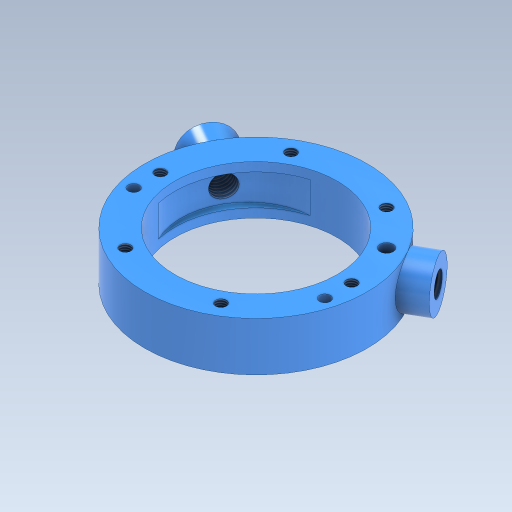
# Autodesk Inventor part: Pump-Motor-CW-Rotation:M Case
Saved by Autodesk Inventor 2024.2 (Build 282272000, 272)
## iProperties
Created: 2025-06-16
Material: Aluminum 6061-AHC
Document SubType Name: Modeling
Density: 2.7 g/cm^3
Appearance: Cyan
Designer: cw
Author: cw
Autodesk Inventor part; units mm, degrees
note: some values were not read from the file. Chosen so that the rebuilt part matches the saved one: direction of "Hole2".
ref_plane "YZ Plane" through (0, 0, 0) normal (1, 0, 0) x (0, 1, 0)
ref_plane "XZ Plane" through (0, 0, 0) normal (0, 1, 0) x (-1, 0, 0)
ref_plane "XY Plane" through (0, 0, 0) normal (0, 0, 1) x (1, 0, 0)
sketch "Sketch1" plane through (0, 0, 0) normal (0, 0, 1) x (1, 0, 0)
  circle A0 centre (0, 0) radius 50
  circle A1 centre (0, 0) radius 36.5
  dimension "d0" = 100
  dimension "d3" = 73
  constraints: 2 centre point, 2 coincident
  measures "d0" diameter of A0
  measures "d3" diameter of A1
extrude "Extrusion1" add sketch "Sketch1" along normal mid plane 22
sketch "Sketch2" plane through (0, 0, 0) normal (0, 0, 1) x (1, 0, 0)
  line L0 (0, 0) -> (51.961524, 30)
  line L1 (51.961524, 30) -> (57.461524, 20.473721)
  line L2 (57.461524, 20.473721) -> (47.740384, 14.861217)
  circle A0 centre (0, 0) radius 50 construction
  line L3 (47.740384, 14.861217) -> (42.240384, 24.387497)
  line L4 (-72.00542, 0) -> (82.032521, 0) construction
  dimension "d4" = 30
  dimension "d5" = 60
  dimension "d6" = 22
  constraints: 8 end point, 3 perpendicular, 1 point on line, 2 other
  measures "d4" angle of L4 L0
  measures "d5" distance from line of L1 L0.start
  measures "d6" diameter of L2 L0
revolve "Revolution1" add sketch "Sketch2" angle 360 about axis through (0, 0, 0) along (0.8660254, 0.5, 0)
mirror "Mirror1" about plane through (0, 0, 0) normal (1, 0, 0) of "Revolution1"
sketch "Sketch3" plane through (51.961524, 30, 0) normal (0.8660254, 0.5, 0) x (0, 0, -1)
  point P0 (0, 0)
hole "Hole1" at (51.961524, 30, 0) direction (-0.8660254, -0.5, 0) diameter 10.106 depth 32.3 tip angle 118 thread size "M12x1.75" class "6H" standard "ISO Metric profile"
sketch "Sketch4" plane through (0, 0, 0) normal (0, 0, 1) x (1, 0, 0)
  line L0 (0, 0) -> (-51.961524, 30) construction
  line L1 (-46.461524, 39.526279) -> (-57.461524, 20.473721) construction
  circle A0 centre (0, 0) radius 36.5
  arc A1 (-10.556856, 34.939988) -> (-35.537346, -8.327488) centre (-8.660254, 5) ccw
  dimension "d15" = 30
  dimension "d16" = 10
  constraints: 4 point on circle, 2 end point, 1 centre point, 1 midpoint, 1 point on line
  measures "d15" radius of A1
  measures "d16" distance of L0.start A1.centre
extrude "Extrusion2" cut sketch "Sketch4" along normal mid plane 14 contours A0 A1
sketch "Sketch5" plane through (-51.961524, 30, 0) normal (-0.8660254, 0.5, 0) x (0, 0, 1)
  point P0 (0, 0)
hole "Hole2" at (-51.961524, 30, 0) direction (0.8660254, -0.5, 0) diameter 10.106 end up to surface thread size "M12x1.75" class "6H" standard "ISO Metric profile"
sketch "Sketch6" plane through (0, 0, -11) normal (0, 0, -1) x (-1, 0, 0)
  circle A0 centre (0, 0) radius 43 construction
  point P0 (-43, 0)
  dimension "d26" = 86
  constraints: 2 horizontal alignment, 1 coincident, 2 other
hole "Hole3" at (43, 0, -11) direction (0, 0, 1) diameter 4.917 end through all thread size "M6x1" class "6H" standard "ISO Metric profile"
pattern_circular "Circular Pattern1" count 6 over 360 about axis through (0, 0, 0) along (0, 0, 1) of "Hole3"
sketch "Sketch7" plane through (0, 0, -11) normal (0, 0, -1) x (-1, 0, 0)
  circle A0 centre (43, 0) radius 2.4585 construction
  circle A1 centre (-43, 0) radius 2.4585 construction
  point P0 (0, 0)
  point P1 (-43, -12)
  point P2 (43, -12)
  dimension "d37" = 12
  constraints: 2 vertical alignment, 1 horizontal alignment
  measures "d37" distance of A1.centre point (-43, -12)
hole "Hole4" at (43, -12, -11) at (-43, -12, -11) direction (0, 0, 1) diameter 5 end through all
sketch "Sketch8" plane through (0, 0, -11) normal (0, 0, -1) x (-1, 0, 0)
  line L0 (80.446134, 0) -> (-80.446134, 0) construction
  line L1 (0, 0) -> (-37.239092, 21.5) construction
  dimension "d45" = 43
  dimension "d46" = 30
  constraints: 2 end point
  measures "d45" distance of L1.start L1.end
  measures "d46" angle of L0 L1
hole "Hole5" at (37.239092, 21.5, -11) direction (0, 0, 1) diameter 6 end through all
body "Solid1"
